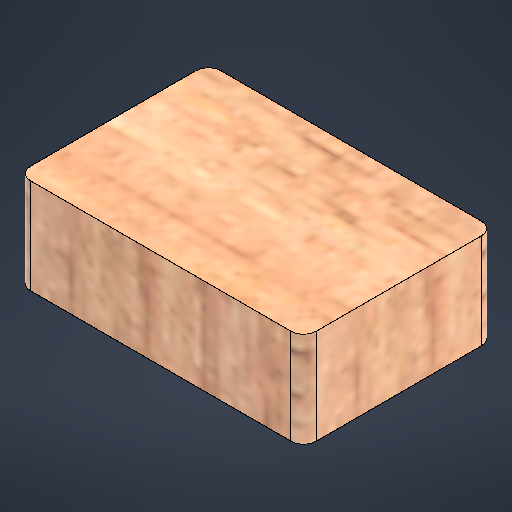
# Autodesk Inventor part: TCSM1-15-005
Saved by Autodesk Inventor 2025.3 (Build 293356000, 356)
## iProperties
Created: 2025-08-26
Part Number: TCSM1-15-005
Material: Wood (Birch)
Document SubType Name: Modeling
Designer: fablabadmin
Density: 0.55 g/cm^3
Appearance: Birch - Natural Polished
Author: fablabadmin
Autodesk Inventor part; units mm, degrees
ref_plane "YZ Plane" through (0, 0, 0) normal (1, 0, 0) x (0, 1, 0)
ref_plane "XZ Plane" through (0, 0, 0) normal (0, 1, 0) x (-1, 0, 0)
ref_plane "XY Plane" through (0, 0, 0) normal (0, 0, 1) x (1, 0, 0)
sketch "Sketch1" plane through (0, 0, 0) normal (0, 1, 0) x (-1, 0, 0)
  line L0 (-22.5, 15) -> (22.5, 15)
  line L1 (22.5, 15) -> (22.5, -15)
  line L2 (22.5, -15) -> (-22.5, -15)
  line L3 (-22.5, -15) -> (-22.5, 15)
  line L4 (-22.5, 15) -> (22.5, -15) construction
  line L5 (22.5, 15) -> (-22.5, -15) construction
  line L6 (31.5, 0) -> (-31.5, 0) construction
  line L7 (0, -21) -> (0, 21) construction
  point P0 (0, 0)
  dimension "d0" = 45
  dimension "d1" = 30
  constraints: 12 end point, 2 midpoint, 2 parallel, 1 horizontal, 1 perpendicular
  measures "d0" distance of L1.end L2.end
  measures "d1" distance of L0.end L1.end
extrude "Extrusion1" add sketch "Sketch1" along normal blind 15
fillet "Fillet1" radius 2 4 edges at (-22.5, 7.5, 15) (-22.5, 7.5, -15) (22.5, 7.5, -15) (22.5, 7.5, 15)
body "Solid1"
